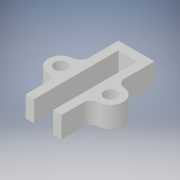
# Autodesk Inventor part: Stand Clamp
Saved by Autodesk Inventor 2019 (Build 230136000, 136)
## iProperties
Created: 2019-11-14
Part Number: Stand Clamp
Material: Generic
Document SubType Name: Modeling
Designer: James
Density: 1 g/cm^3
Appearance: Default
Author: James
Autodesk Inventor part; units mm, degrees
ref_plane "YZ Plane" through (0, 0, 0) normal (1, 0, 0) x (0, 1, 0)
ref_plane "XZ Plane" through (0, 0, 0) normal (0, 1, 0) x (-1, 0, 0)
ref_plane "XY Plane" through (0, 0, 0) normal (0, 0, 1) x (1, 0, 0)
sketch "Sketch1" plane through (0, 0, 0) normal (0, 1, 0) x (-1, 0, 0)
  line L0 (2.25, 10) -> (-2.25, 10)
  line L1 (-2.25, 10) -> (-2.25, -10)
  line L2 (-2.25, -10) -> (2.25, -10)
  line L3 (2.25, -10) -> (2.25, 10)
  line L4 (4.25, 10) -> (-4.25, 10)
  line L5 (-4.25, -12) -> (4.25, -12)
  circle A0 centre (5.9, 0) radius 1.5
  circle A1 centre (-5.9, 0) radius 1.5
  arc A2 (-4.25, 2.5055) -> (-4.25, -2.5055) centre (-5.9, 0) ccw
  arc A3 (4.25, -2.5055) -> (4.25, 2.5055) centre (5.9, 0) ccw
  line L6 (4.25, -12) -> (4.25, -2.5055)
  line L7 (4.25, 2.5055) -> (4.25, 10)
  line L8 (-4.25, 10) -> (-4.25, 2.5055)
  line L9 (-4.25, -2.5055) -> (-4.25, -12)
  point P0 (0, 0)
  point P1 (0, -12)
  point P2 (0, -10)
  point P3 (2.25, 0)
  dimension "d0" = 4.5
  dimension "d1" = 20
  dimension "d2" = 5.9
  dimension "d3" = 11.8
  dimension "d4" = 3
  dimension "d5" = 3
  dimension "d6" = 6
  dimension "d7" = 6
  dimension "d8" = 2
  dimension "d9" = 2
  dimension "d10" = 2
  dimension "d11" = 2
  constraints: 20 end point, 7 parallel, 4 centre point, 4 point on circle, 3 horizontal alignment, 3 midpoint, 3 perpendicular, 2 coincident, 2 horizontal, 2 vertical alignment, 1 point on line
  measures "d0" distance between parallel lines of L1 L3
  measures "d1" distance of L2.end L0.start
  measures "d2" distance of point (0, 0) A0.centre
  measures "d3" distance of A1.centre A0.centre
  measures "d4" diameter of A0
  measures "d5" diameter of A1
  measures "d6" diameter of A2
  measures "d7" diameter of A3
  measures "d8" distance between parallel lines of L7 L3
  measures "d9" distance between parallel lines of L6 L3
  measures "d10" distance between parallel lines of L1 L8
  measures "d11" distance between parallel lines of L2 L5
extrude "Extrusion1" add sketch "Sketch1" along normal blind 5 contours L4 L7 A3 L6 L5 L9 A2 L8 L1 L2 L3
fillet "Fillet1" radius 2 4 edges at (4.25, 2.5, 2.5055) (-4.25, 2.5, 2.5055) (-4.25, 2.5, -2.5055) (4.25, 2.5, -2.5055)
body "Solid1"
